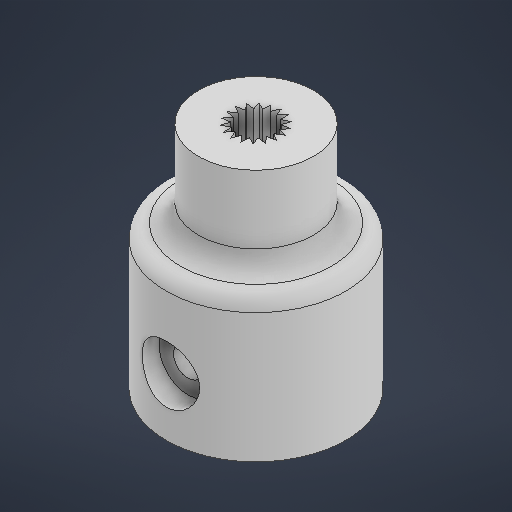
# Autodesk Inventor part: 가변저항-조향 연결
Saved by Autodesk Inventor 2026.2 (Build 302298000, 298)
## iProperties
Created: 2025-11-20
Part Number: 가변저항-조향 연결
Material: 일반
Document SubType Name: Modeling
Designer: PC
Density: 1 g/cm^3
Appearance: 기본값
Author: PC
Autodesk Inventor part; units mm, degrees
sketch "스케치1" plane through (0, 0, 0) normal (0, 1, 0) x (-1, 0, 0)
  line L0 (17.5, 0) -> (-17.5, 0) projected
  line L1 (0, -17.5) -> (0, 17.5) projected
  circle A0 centre (0, 0) radius 5.25
  circle A1 centre (0, 0) radius 12.5
  dimension "d0" = 10.5
  dimension "d1" = 25
  constraints: 2 centre point, 2 coincident
  measures "d0" diameter of A0
  measures "d1" diameter of A1
extrude "돌출1" add sketch "스케치1" along normal blind 20 contours A1 L1 A0 L0 | L0 A0 L1 A1 | L1 A0 L0 A1 | A1 L0 A0 L1
ref_plane "작업 평면1" through (0, 0, 12.5) normal (0, 0, 1) x (1, 0, 0)
sketch "스케치2" plane through (0, 0, 12.5) normal (0, 0, 1) x (1, 0, 0)
  line L0 (0, 0) -> (0, 8)
  circle A0 centre (0, 8) radius 2
  dimension "d5" = 8
  dimension "d6" = 4
  constraints: 2 end point, 1 centre point, 1 coincident, 1 vertical
  measures "d5" distance of L0.start L0.end
  measures "d6" diameter of A0
extrude "돌출2" cut sketch "스케치2" against normal blind 40
sketch "스케치3" plane through (0, 0, 12.5) normal (0, 0, 1) x (1, 0, 0)
  line L0 (0, 0) -> (0, 8)
  circle A0 centre (0, 8) radius 4
  point P0 (0, 6)
  point P1 (0, 10)
  dimension "d10" = 8
  dimension "d11" = 8
  constraints: 2 end point, 2 vertical alignment, 1 centre point, 1 coincident, 1 vertical
  measures "d10" distance of L0.start L0.end
  measures "d11" diameter of A0
extrude "돌출3" cut sketch "스케치3" against normal blind 3
ref_plane "작업 평면2" through (0, 0, -12.5) normal (0, 0, 1) x (1, 0, 0)
sketch "스케치4" plane through (0, 0, -12.5) normal (0, 0, 1) x (1, 0, 0)
  line L0 (0, 0) -> (0, 8)
  circle A0 centre (0, 8) radius 2 projected
  line L1 (0, 8) -> (-2.05, 4.4493)
  line L2 (0, 8) -> (2.05, 4.4493)
  line L3 (2.05, 4.4493) -> (-2.05, 4.4493)
  line L4 (4.1, 8) -> (2.05, 4.4493)
  line L5 (2.05, 11.5507) -> (4.1, 8)
  line L6 (-2.05, 11.5507) -> (2.05, 11.5507)
  line L7 (-4.1, 8) -> (-2.05, 11.5507)
  line L8 (-2.05, 4.4493) -> (-4.1, 8)
  point P0 (2.05, 4.4493)
  point P1 (4.1, 8)
  point P2 (2.05, 11.5507)
  point P3 (-2.05, 11.5507)
  point P4 (-4.1, 8)
  point P5 (-2.05, 4.4493)
  dimension "d15" = 8
  dimension "d16" = 4.1
  dimension "d17" = 30
  dimension "d20" = 360
  constraints: 18 end point, 1 horizontal, 1 symmetric about line, 1 vertical, 19 other
  measures "d15" distance of L0.start L0.end
  measures "d16" distance of L1.start L1.end
  measures "d17" angle of L0 L1
extrude "돌출4" cut sketch "스케치4" along normal blind 4
fillet "모깎기1" radius 2 1 edges at (12.5, 20, 0)
sketch "스케치6" plane through (0, 0, 0) normal (0, 0, 1) x (1, 0, 0)
  line L0 (8, 32) -> (8, 22.5)
  line L1 (-15.1828, 0) -> (17.5971, 0) projected
  line L2 (0, -6.4) -> (0, 38.4) projected
  arc A0 (12.5, 18) -> (10.5, 20) centre (10.5, 18) ccw projected
  arc A1 (8, 22.5) -> (10.5, 20) centre (10.5, 22.5) ccw
  line L3 (-10.5, 20) -> (10.5, 20) projected
  line L4 (8, 32) -> (0, 32)
  point P0 (0, 0)
  point P1 (0, 20)
  dimension "d24" = 8
  dimension "d26" = 12
  constraints: 4 end point, 2 point on circle, 2 tangent, 1 centre point, 1 perpendicular, 1 point on line, 1 vertical
  measures "d24" distance between parallel lines of L2 L0
  measures "d26" distance from line of L0.start L3
revolve "회전1" add sketch "스케치6" angle 360 about axis through (0, -10, 0) along (0, 1, 0)
ref_plane "작업 평면3" through (0, 0, 8) normal (0, 0, 1) x (1, 0, 0)
sketch "스케치8" plane through (0, 32, 0) normal (0, 1, 0) x (1, 0, 0)
  circle A0 centre (0, 0) radius 2.5
  line L0 (0, 3.5) -> (-0.4341, 2.462)
  line L1 (-0.4341, 2.462) -> (0, 3.5)
  line L2 (0, 17.5005) -> (0, -17.5027) projected
  line L3 (0.4341, 2.462) -> (0, 3.5)
  line L4 (-1.1971, 3.2889) -> (-1.25, 2.1651)
  line L5 (-0.4341, 2.462) -> (-1.1971, 3.2889)
  line L6 (-2.2498, 2.6812) -> (-1.9151, 1.607)
  line L7 (-1.25, 2.1651) -> (-2.2498, 2.6812)
  line L8 (-3.0311, 1.75) -> (-2.3492, 0.8551)
  line L9 (-1.9151, 1.607) -> (-3.0311, 1.75)
  line L10 (-3.4468, 0.6078) -> (-2.5, 0)
  line L11 (-2.3492, 0.8551) -> (-3.4468, 0.6078)
  line L12 (-3.4468, -0.6078) -> (-2.3492, -0.8551)
  line L13 (-2.5, 0) -> (-3.4468, -0.6078)
  line L14 (-3.0311, -1.75) -> (-1.9151, -1.607)
  line L15 (-2.3492, -0.8551) -> (-3.0311, -1.75)
  line L16 (-2.2498, -2.6812) -> (-1.25, -2.1651)
  line L17 (-1.9151, -1.607) -> (-2.2498, -2.6812)
  line L18 (-1.1971, -3.2889) -> (-0.4341, -2.462)
  line L19 (-1.25, -2.1651) -> (-1.1971, -3.2889)
  line L20 (0, -3.5) -> (0.4341, -2.462)
  line L21 (-0.4341, -2.462) -> (0, -3.5)
  line L22 (1.1971, 3.2889) -> (1.25, 2.1651)
  line L23 (0.4341, 2.462) -> (1.1971, 3.2889)
  line L24 (2.2498, 2.6812) -> (1.9151, 1.607)
  line L25 (1.25, 2.1651) -> (2.2498, 2.6812)
  line L26 (3.0311, 1.75) -> (2.3492, 0.8551)
  line L27 (1.9151, 1.607) -> (3.0311, 1.75)
  line L28 (3.4468, 0.6078) -> (2.5, 0)
  line L29 (2.3492, 0.8551) -> (3.4468, 0.6078)
  line L30 (3.4468, -0.6078) -> (2.3492, -0.8551)
  line L31 (2.5, 0) -> (3.4468, -0.6078)
  line L32 (3.0311, -1.75) -> (1.9151, -1.607)
  line L33 (2.3492, -0.8551) -> (3.0311, -1.75)
  line L34 (2.2498, -2.6812) -> (1.25, -2.1651)
  line L35 (1.9151, -1.607) -> (2.2498, -2.6812)
  line L36 (1.1971, -3.2889) -> (0.4341, -2.462)
  line L37 (1.25, -2.1651) -> (1.1971, -3.2889)
  line L38 (0, 2.5) -> (0, 3.5)
  point P0 (-2.5, 0)
  point P1 (2.5, 0)
  dimension "d33" = 5
  dimension "d36" = 180
  dimension "d38" = 1
  constraints: 76 end point, 25 symmetric about line, 2 coincident, 2 point on circle, 2 point on line, 1 centre point, 1 collinear, 46 other
  measures "d33" diameter of A0
  measures "d38" distance of L38.start L0.start
extrude "돌출6" cut sketch "스케치8" against normal up to surface (12 mm away)
